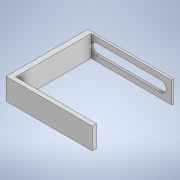
# Autodesk Inventor part: Suporte prensas coletor
Saved by Autodesk Inventor 2021 (Build 250183000, 183)
## iProperties
Created: 2020-09-23
Part Number: Suporte prensas coletor
Material: Genérico
Document SubType Name: Modeling
Designer: rapha
Density: 1 g/cm^3
Appearance: Padrão
Author: rapha
Autodesk Inventor part; units mm, degrees
ref_plane "YZ Plane" through (0, 0, 0) normal (1, 0, 0) x (0, 1, 0)
ref_plane "XZ Plane" through (0, 0, 0) normal (0, 1, 0) x (-1, 0, 0)
ref_plane "XY Plane" through (0, 0, 0) normal (0, 0, 1) x (1, 0, 0)
sketch "Esboço1" plane through (0, 0, 0) normal (0, 0, 1) x (1, 0, 0)
  line L0 (0, 0) -> (40, 0)
  line L1 (40, 0) -> (40, 10)
  line L2 (40, 10) -> (0, 10)
  line L3 (0, 10) -> (0, 0)
  dimension "d0" = 40
  dimension "d1" = 10
  constraints: 8 end point, 2 parallel, 1 horizontal, 1 perpendicular
  measures "d0" distance of L2.end L1.end
  measures "d1" distance of L1.end L0.end
extrude "Extrusão1" add sketch "Esboço1" along normal blind 1
sketch "Esboço2" plane through (0, 0, 1) normal (0, 0, 1) x (1, 0, 0)
  line L0 (5, 5) -> (35, 5) construction
  line L1 (5, 2.5) -> (35, 2.5)
  line L2 (35, 7.5) -> (5, 7.5)
  arc A0 (5, 7.5) -> (5, 2.5) centre (5, 5) ccw
  arc A1 (35, 2.5) -> (35, 7.5) centre (35, 5) ccw
  point P0 (0, 0)
  point P1 (20, 5)
  dimension "d4" = 30
  dimension "d5" = 5
  constraints: 8 end point, 4 point on circle, 4 tangent, 2 centre point, 1 horizontal, 1 midpoint, 1 parallel
  measures "d4" distance of L0.start L0.end
  measures "d5" diameter of A1
extrude "Extrusão2" cut sketch "Esboço2" against normal blind 1
sketch "Esboço3" plane through (0, 0, 1) normal (0, 0, 1) x (1, 0, 0)
  line L0 (40, 10) -> (0, 10) projected
  line L1 (0, 0) -> (40, 0) projected
  line L2 (0, 10) -> (2.5, 10)
  line L3 (2.5, 10) -> (2.5, 0)
  line L4 (2.5, 0) -> (0, 0)
  line L5 (0, 0) -> (0, 10)
  dimension "d8" = 2.5
  constraints: 8 end point, 2 parallel, 1 horizontal, 1 perpendicular, 1 point on line
  measures "d8" distance of L3.end L4.end
extrude "Extrusão3" add sketch "Esboço3" along normal blind 35
sketch "Esboço4" plane through (0, 0, 36) normal (0, 0, 1) x (1, 0, 0)
  line L0 (0, 10) -> (0, 0) projected
  line L1 (0, 10) -> (40.017, 10)
  line L2 (40.017, 10) -> (40.017, 0)
  line L3 (40.017, 0) -> (0, 0)
  line L4 (0, 0) -> (0, 10)
  constraints: 8 end point, 2 parallel, 1 horizontal, 1 perpendicular
extrude "Extrusão4" add sketch "Esboço4" along normal blind 2
